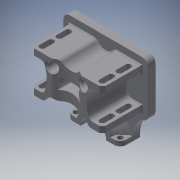
# Autodesk Inventor part: x-carriage
Saved by Autodesk Inventor 2018 (Build 220112000, 112)
## iProperties
Created: 2017-10-14
Part Number: x-carriage
Material: Generic
Document SubType Name: Modeling
Designer: Jurjen
Density: 1 g/cm^3
Appearance: Default
Author: Jurjen
Autodesk Inventor part; units mm, degrees
ref_plane "YZ Plane" through (0, 0, 0) normal (1, 0, 0) x (0, 1, 0)
ref_plane "XZ Plane" through (0, 0, 0) normal (0, 1, 0) x (-1, 0, 0)
ref_plane "XY Plane" through (0, 0, 0) normal (0, 0, 1) x (1, 0, 0)
sketch "Sketch1" plane through (0, 0, 0) normal (0, 0, 1) x (1, 0, 0)
  line L0 (-27, 20) -> (27, 20)
  line L1 (27, 20) -> (27, -15)
  line L2 (27, -15) -> (-27, -15)
  line L3 (-27, -15) -> (-27, 20)
  point P0 (0, 0)
  point P1 (0, 20)
  point P2 (-27, 2.5)
  dimension "d0" = 54
  dimension "d69" = 20
  dimension "d70" = 15
  constraints: 8 end point, 2 midpoint, 2 parallel, 1 horizontal, 1 perpendicular, 1 vertical alignment
  measures "d0" distance between parallel lines of L1 L3
  measures "d69" distance from line of L0 point (0, 0)
  measures "d70" distance from line of point (0, 0) L2
extrude "Extrusion1" add sketch "Sketch1" along normal mid plane 5
sketch "Sketch2" plane through (0, 0, 2.5) normal (0, 0, 1) x (1, 0, 0)
  circle A0 centre (10, 10) radius 1.6
  circle A1 centre (-10, 10) radius 1.6
  circle A2 centre (-10, -10) radius 1.6
  circle A3 centre (10, -10) radius 1.6
  line L0 (-10, 10) -> (10, 10) construction
  line L1 (-10, -10) -> (-10, 10) construction
  point P0 (0, 0)
  point P1 (0, 10)
  point P2 (-10, 0)
  dimension "d4" = 20
  dimension "d5" = 20
  dimension "d6" = 3.2
  constraints: 4 centre point, 4 end point, 3 equal radius, 3 horizontal alignment, 3 vertical alignment, 2 midpoint, 1 horizontal, 1 vertical
  measures "d4" distance of L0.end L0.start
  measures "d5" distance of L1.start L0.start
  measures "d6" diameter of A1
extrude "Extrusion2" cut sketch "Sketch2" against normal up to next
fillet "Fillet1" radius 4 4 edges at (-27, 20, 0) (-27, -15, 0) (27, -15, 0) (27, 20, 0)
sketch "Sketch3" plane through (0, 0, 2.5) normal (0, 0, 1) x (1, 0, 0)
  line L0 (-23, -15) -> (23, -15) projected
  arc A0 (8.15, -30) -> (-8.15, -30) centre (0, -30) ccw
  line L1 (17.15, -30) -> (8.15, -30)
  arc A1 (23, -15) -> (17.15, -30) centre (34.9437, -28.2988) ccw
  line L2 (0, -30) -> (0, 0) construction
  line L3 (-17.15, -30) -> (-8.15, -30)
  arc A2 (-17.15, -30) -> (-23, -15) centre (-34.9437, -28.2988) ccw
  dimension "d10" = 30
  dimension "d12" = 9
  dimension "d13" = 16.3
  constraints: 6 end point, 6 point on circle, 3 centre point, 3 symmetric about line, 1 horizontal, 1 horizontal alignment, 1 vertical, 1 vertical alignment, 1 other
  measures "d10" distance of L2.start L2.end
  measures "d12" distance of L1.start L1.end
  measures "d13" diameter of A0
extrude "Extrusion3" add sketch "Sketch3" against normal up to surface (5 mm away)
sketch "Sketch4" plane through (0, 0, 2.5) normal (0, 0, 1) x (1, 0, 0)
  arc A0 (8.15, -30) -> (-8.15, -30) centre (0, -30) ccw projected
  arc A1 (6.25, -30) -> (-6.25, -30) centre (0, -30) ccw
  line L0 (-6.25, -30) -> (-17.15, -30)
  arc A2 (-17.15, -30) -> (-23, -15) centre (-34.9437, -28.2988) ccw projected
  line L1 (17.15, -30) -> (8.15, -30) projected
  line L2 (17.15, -30) -> (6.25, -30)
  arc A3 (8.15, -30) -> (-8.15, -30) centre (0, -30) ccw
  point P0 (0, 0)
  dimension "d16" = 12.5
  constraints: 6 point on circle, 4 end point, 2 centre point, 2 coincident, 2 point on line, 1 collinear, 1 horizontal alignment
  measures "d16" diameter of A1
extrude "Extrusion4" add sketch "Sketch4" along normal blind 3.8 and the other way blind 1.8
sketch "Sketch5" plane through (0, 0, 2.5) normal (0, 0, 1) x (1, 0, 0)
  arc A0 (27, 16) -> (23, 20) centre (23, 16) ccw projected
  line L0 (23, 20) -> (-23, 20) projected
  arc A1 (-23, 20) -> (-27, 16) centre (-23, 16) ccw projected
  line L1 (-27, 16) -> (-27, -11) projected
  arc A2 (-27, -11) -> (-23, -15) centre (-23, -11) ccw projected
  arc A3 (-17.15, -30) -> (-23, -15) centre (-34.9437, -28.2988) ccw projected
  line L2 (-8.15, -30) -> (-17.15, -30) projected
  arc A4 (8.15, -30) -> (-8.15, -30) centre (0, -30) ccw projected
  line L3 (17.15, -30) -> (8.15, -30) projected
  arc A5 (23, -15) -> (17.15, -30) centre (34.9437, -28.2988) ccw projected
  arc A6 (23, -15) -> (27, -11) centre (23, -11) ccw projected
  line L4 (27, -11) -> (27, 16) projected
  circle A7 centre (-10, -10) radius 1.6 projected
  circle A8 centre (10, 10) radius 1.6 projected
  circle A9 centre (-10, 10) radius 1.6 projected
  circle A10 centre (10, -10) radius 1.6 projected
  arc A11 (23, -15) -> (17.15, -30) centre (34.9437, -28.2988) ccw projected
  line L5 (17.1161, -27) -> (7.5778, -27)
  line L6 (-7.5778, -27) -> (-17.1161, -27)
  point P0 (0, 0)
  dimension "d21" = 3
  constraints: 4 end point, 4 point on circle, 2 point on line, 1 horizontal
  measures "d21" distance between parallel lines of L3 L5
extrude "Extrusion5" add sketch "Sketch5" along normal up to surface (3.8 mm away) contours A5 L3 A4 L5 | A4 L2 A3 L6
sketch "Sketch6" plane through (0, 0, 6.3) normal (0, 0, 1) x (1, 0, 0)
  arc A0 (8.15, -30) -> (-8.15, -30) centre (0, -30) ccw projected
  arc A1 (8.15, -30) -> (-8.15, -30) centre (0, -30) ccw
  arc A2 (11.15, -30) -> (-11.15, -30) centre (0, -30) ccw
  arc A3 (6.25, -30) -> (-6.25, -30) centre (0, -30) ccw projected
  line L0 (-6.25, -30) -> (-17.15, -30) projected
  line L1 (-6.25, -30) -> (-17.15, -30)
  line L2 (6.25, -30) -> (12.2947, -30)
  point P0 (0, 0)
  dimension "d24" = 3
  constraints: 6 point on circle, 4 end point, 4 point on line, 2 centre point, 2 coincident, 2 horizontal
  measures "d24" radial gap between concentric circles of A2 A1
extrude "Extrusion6" add sketch "Sketch6" along normal blind 4 contours A0 L0 A2 L2
sketch "Sketch9" plane through (0, 0, 6.3) normal (0, 0, 1) x (1, 0, 0)
  arc A0 (-10.7388, -27) -> (-11.15, -30) centre (0, -30) ccw projected
  line L0 (-17.1161, -27) -> (-10.7388, -27) projected
  arc A1 (-17.15, -30) -> (-17.1161, -27) centre (-34.9437, -28.2988) ccw projected
  line L1 (-11.15, -30) -> (-17.15, -30) projected
  arc A2 (11.15, -30) -> (10.7388, -27) centre (0, -30) ccw projected
  line L2 (11.15, -30) -> (17.15, -30) projected
  arc A3 (17.1161, -27) -> (17.15, -30) centre (34.9437, -28.2988) ccw projected
  line L3 (10.7388, -27) -> (17.1161, -27) projected
  point P0 (0, 0)
extrude "Extrusion7" add sketch "Sketch9" along normal up to surface (4 mm away)
sketch "Sketch10" plane through (0, 0, 6.3) normal (0, 0, -1) x (-1, 0, 0)
  line L0 (10.7388, -27) -> (7.5778, -27) projected
  arc A0 (10.7388, -27) -> (-10.7388, -27) centre (0, -30) ccw projected
  line L1 (-7.5778, -27) -> (-10.7388, -27) projected
  arc A1 (7.5778, -27) -> (-7.5778, -27) centre (0, -30) ccw projected
  point P0 (0, 0)
extrude "Extrusion8" add sketch "Sketch10" along normal up to surface (3.8 mm away)
chamfer "Chamfer1" distance 5 angle 45 1 edges at (0, -18.85, 2.5)
fillet "Fillet2" radius 4 2 edges at (17.07, -28.5007, 10.3) (-17.07, -28.5007, 10.3)
fillet "Fillet3" radius 4 2 edges at (0, -18.85, 7.5) (0, -13.85, 2.5)
sketch "Sketch13" plane through (-17.15, -30, -2.5) normal (0, -1, 0) x (1, 0, 0)
  circle A0 centre (3, 9.8) radius 1.6
  circle A1 centre (31.3, 9.8) radius 1.6
  line L0 (0, 0) -> (0, 8.8) projected
  line L1 (9, 12.8) -> (4.0149, 12.8) projected
  line L2 (34.3, 8.8) -> (34.3, 0) projected
  point P0 (17.15, 2.5)
  dimension "d45" = 3.2
  dimension "d46" = 3
  dimension "d47" = 3
  dimension "d48" = 3
  constraints: 2 centre point, 1 equal radius, 1 horizontal alignment
  measures "d45" diameter of A0
  measures "d46" distance from line of A0.centre L0
  measures "d47" distance from line of L1 A0.centre
  measures "d48" distance from line of A1.centre L2
extrude "Extrusion10" cut sketch "Sketch13" against normal up to next
sketch "Sketch17" plane through (0, 0, 2.5) normal (0, 0, 1) x (1, 0, 0)
  line L0 (-13.1229, -10.9) -> (-23, -10.9)
  line L1 (-23, -10.9) -> (-23, -6.9)
  line L2 (-23, -6.9) -> (-14, -6.9)
  line L3 (-14, -6.9) -> (-14, -4.9)
  line L4 (-14, 11.2) -> (-23, 11.2)
  circle A0 centre (-10, 10) radius 1.6 projected
  circle A1 centre (-10, 10) radius 3
  circle A2 centre (-10, -10) radius 1.6 projected
  arc A3 (-7.3604, -8.104) -> (-13.1229, -10.9) centre (-10, -10) ccw
  line L5 (-23, 15.2) -> (-6, 15.2)
  line L6 (-23, 11.2) -> (-23, 15.2)
  line L7 (0, 0) -> (0, 11.3763) construction
  arc A4 (-6, 15.2) -> (0, 11.3763) centre (-0.0763, 17.8758) ccw
  arc A5 (0, -6.9) -> (-7.3604, -8.104) centre (0, -30) ccw
  line L8 (0, -6.9) -> (0, 0) construction
  arc A6 (-7, -1.7545) -> (-7, 6.0545) centre (-14.1224, 2.15) ccw
  arc A7 (0, -0.9) -> (-7, -1.7545) centre (0, -30) ccw
  line L9 (13.1229, -10.9) -> (23, -10.9)
  line L10 (23, -10.9) -> (23, -6.9)
  line L11 (23, -6.9) -> (14, -6.9)
  line L12 (14, 11.2) -> (23, 11.2)
  circle A8 centre (10, 10) radius 3
  arc A9 (13.1229, -10.9) -> (7.3604, -8.104) centre (10, -10) ccw
  line L13 (23, 15.2) -> (6, 15.2)
  line L14 (23, 11.2) -> (23, 15.2)
  arc A10 (0, 11.3763) -> (6, 15.2) centre (0.0763, 17.8758) ccw
  arc A11 (7.3604, -8.104) -> (0, -6.9) centre (0, -30) ccw
  arc A12 (7, 6.0545) -> (7, -1.7545) centre (14.1224, 2.15) ccw
  arc A13 (7, -1.7545) -> (0, -0.9) centre (0, -30) ccw
  arc A14 (14.6749, -27) -> (-14.6749, -27) centre (0, -30) ccw projected
  arc A15 (-7, 6.0545) -> (0, 4.9807) centre (0.8793, 34.0674) ccw
  arc A16 (0, 4.9807) -> (7, 6.0545) centre (-0.8793, 34.0674) ccw
  arc A17 (-14, -4.9) -> (-14, 9.2) centre (-32.7162, 2.15) ccw
  arc A18 (14, 9.2) -> (14, -4.9) centre (32.7162, 2.15) ccw
  line L15 (14, -6.9) -> (14, -4.9)
  line L16 (14, 9.2) -> (14, 11.2)
  line L17 (-14, 9.2) -> (-14, 11.2)
  line L18 (-14, -4.9) -> (-14, 9.2) construction
  point P0 (0, 8.6643)
  point P1 (-14, 2.15)
  point P2 (-6, 2.15)
  point P3 (-12.7162, 2.15)
  dimension "d71" = 6
  dimension "d72" = 6.5
  dimension "d73" = 4
  dimension "d75" = 4
  dimension "d76" = 17
  dimension "d77" = 18.1
  dimension "d78" = 14
  dimension "d80" = 6.5
  dimension "d81" = 9
  dimension "d82" = 11.2
  dimension "d98" = 6
  dimension "d99" = 6
  dimension "d100" = 7
  dimension "d103" = 29.1
  dimension "d104" = 20
  dimension "d105" = 2
  dimension "d106" = 2
  constraints: 38 end point, 30 point on circle, 22 symmetric about line, 16 centre point, 9 perpendicular, 5 point on line, 3 vertical, 3 vertical alignment, 2 coincident, 2 concentric, 2 horizontal alignment, 8 other
  measures "d71" diameter of A1
  measures "d72" diameter of A3
  measures "d73" distance between parallel lines of L0 L2
  measures "d75" distance between parallel lines of L5 L4
  measures "d76" distance of L5.start L5.end
  measures "d77" distance of L2.end L4.start
  measures "d78" distance from line of L7.start L3
  measures "d80" radius of A4
  measures "d81" distance between parallel lines of L6 L3
  measures "d82" distance from line of L7.start L4
  measures "d98" distance of L8.start A7.start
  measures "d99" distance from line of L7 point (-6, 2.15)
  measures "d100" distance from line of L7 A6.end
  measures "d103" radius of A15
  measures "d104" radius of A17
  measures "d105" distance of L2.end L3.end
  measures "d106" distance of L4.start L17.start
extrude "Extrusion13" add sketch "Sketch17" along normal blind 25 contours L0 L1 L2 L3 A17 L17 L4 L6 L5 A4 A10 L13 L14 L12 L16 A18 L15 L11 L10 L9 A9 A11 A5 A3
fillet "Fillet6" radius 3 13 edges at (-14, 11.2, 15) (-14, 9.2, 15) (-14, -4.9, 15) (-14, -6.9, 15) (6, 15.2, 15) (-6, 15.2, 15) (-7.3604, -8.104, 15) (7.3604, -8.104, 15) (13.1229, -10.9, 15) (-13.1229, -10.9, 15) (14, 11.2, 15) (14, -4.9, 15) (14, -6.9, 15)
sketch "Sketch18" plane through (-23, -10.9, 2.5) normal (0, -1, 0) x (1, 0, 0)
  line L0 (7.1134, 25) -> (7.1134, 0) projected
  line L1 (0, 25) -> (7.1134, 25) projected
  line L2 (0, 0) -> (0, 25) projected
  line L3 (7.1134, 0) -> (0, 0) projected
  line L4 (2, 23) -> (5.5, 23)
  line L5 (5.5, 23) -> (5.5, 14)
  line L6 (5.5, 14) -> (2, 14)
  line L7 (2, 14) -> (2, 23)
  line L8 (2, 12) -> (5.5, 12)
  line L9 (5.5, 12) -> (5.5, 3)
  line L10 (5.5, 3) -> (2, 3)
  line L11 (2, 3) -> (2, 12)
  point P0 (23, -2.5)
  dimension "d110" = 3.5
  dimension "d111" = 2
  dimension "d112" = 2
  dimension "d113" = 9
  dimension "d114" = 2
  dimension "d115" = 9
  constraints: 16 end point, 4 parallel, 2 horizontal, 2 perpendicular, 2 vertical alignment, 1 point on line
  measures "d110" distance of L4.start L4.end
  measures "d111" distance between parallel lines of L2 L7
  measures "d112" distance between parallel lines of L1 L4
  measures "d113" distance between parallel lines of L4 L6
  measures "d114" distance between parallel lines of L6 L8
  measures "d115" distance between parallel lines of L10 L8
extrude "Extrusion14" cut sketch "Sketch18" against normal through all contours L4 L5 L6 L7 | L8 L9 L10 L11
chamfer "Chamfer2" distance 1 angle 45 16 edges at (-17.5, -8.9, 25.5) (-21, -8.9, 25.5) (-17.5, -8.9, 14.5) (-21, -8.9, 14.5) (-21, -8.9, 5.5) (-21, -8.9, 16.5) (-17.5, -8.9, 5.5) (-17.5, -8.9, 16.5) (-17.5, 13.2, 16.5) (-17.5, 13.2, 5.5) (-17.5, 13.2, 14.5) (-17.5, 13.2, 25.5) (-21, 13.2, 5.5) (-21, 13.2, 16.5) (-21, 13.2, 25.5) (-21, 13.2, 14.5)
mirror "Mirror2" about plane through (0, 0, 0) normal (1, 0, 0) of "Extrusion14", "Chamfer2"
chamfer "Chamfer4" distance 2 angle 45 4 edges at (23, -8.9, 27.5) (23, 13.2, 27.5) (-23, -8.9, 27.5) (-23, 13.2, 27.5)
chamfer "Chamfer5" distance 0.7 angle 45 32 edges at (-19.4433, -10.9, 2.5) (-14.1581, -10.3519, 2.5) (-11.0447, -6.9225, 2.5) (-7.0827, -7.7127, 2.5) (0, -6.9, 2.5) (7.0827, -7.7127, 2.5) (11.0447, -6.9225, 2.5) (14.1581, -10.3519, 2.5) (19.4433, -10.9, 2.5) (-23, -8.9, 2.5) (-19.9142, -6.9, 2.5) (-15.1035, -6.3545, 2.5) (-13.9989, -4.8974, 2.5) (-12.7162, 2.15, 2.5) (-13.9989, 9.1974, 2.5) (-15.1035, 10.6545, 2.5) (-19.9142, 11.2, 2.5) (-15.3472, 15.2, 2.5) (-6.3485, 14.8811, 2.5) (-2.9583, 12.0497, 2.5) (-23, 13.2, 2.5) (15.3472, 15.2, 2.5) (6.3485, 14.8811, 2.5) (2.9583, 12.0497, 2.5) (12.7162, 2.1615, 2.5) (13.9989, -4.8974, 2.5) (15.1035, -6.3545, 2.5) (19.9142, -6.9, 2.5) (15.0964, 10.6495, 2.5) (19.9142, 11.2, 2.5) (23, 13.2, 2.5) (23, -8.9, 2.5)
sketch "Sketch19" plane through (-21, -10.9, 27.5) normal (0, -1, 0) x (1, 0, 0)
  line L0 (0, 0) -> (4.1716, 0) projected
  line L1 (7.0081, 0) -> (4.1716, 0) projected
  line L2 (7.0081, 0) -> (7.0081, 0) projected
  line L3 (7.0081, 0) -> (7.0081, 0) projected
  line L4 (6.9941, 0) -> (7.0081, 0) projected
  line L5 (4.1716, 0) -> (6.9941, 0) projected
  line L6 (4.1716, 0) -> (0, 0) projected
  line L7 (0, 0) -> (5.1134, 0) projected
  line L8 (7.9389, 0) -> (5.1134, 0) projected
  line L9 (7.9389, 0) -> (12.7637, 0) projected
  line L10 (15.1514, 0) -> (12.7637, 0) projected
  line L11 (15.1514, 0) -> (26.8486, 0) projected
  line L12 (29.2363, 0) -> (26.8486, 0) projected
  line L13 (29.2363, 0) -> (34.0611, 0) projected
  line L14 (36.8866, 0) -> (34.0611, 0) projected
  line L15 (36.8866, 0) -> (42, 0) projected
  line L16 (42, 0) -> (37.8284, 0) projected
  line L17 (35.0059, 0) -> (37.8284, 0) projected
  line L18 (34.9919, 0) -> (35.0059, 0) projected
  line L19 (34.9919, 0) -> (35, 0) projected
  line L20 (37.8284, 0) -> (35, 0) projected
  line L21 (37.8284, 0) -> (42, 0) projected
  line L22 (42, 0) -> (28.6944, 0) projected
  line L23 (26.2887, 0) -> (28.6944, 0) projected
  line L24 (26.2887, 0) -> (21, 0) projected
  line L25 (21, 0) -> (15.7113, 0) projected
  line L26 (13.3056, 0) -> (15.7113, 0) projected
  line L27 (13.3056, 0) -> (0, 0) construction
  line L28 (14, 0) -> (21, 0) projected
  line L29 (21, 0) -> (28, 0) projected
  line L30 (28, 0) -> (28, 0) projected
  line L31 (28, 0) -> (14, 0) projected
  line L32 (14, 0) -> (14, 0) projected
  arc A0 (11.7122, 0) -> (30.2878, 0) centre (21, 11.7786) ccw
  line L33 (11.7122, 0) -> (30.2878, 0)
  line L34 (7.0081, 0) -> (4.1716, 0) projected
  point P0 (21, -27.5)
  point P1 (15, 0)
  point P2 (7, 0)
  point P3 (27, 0)
  point P4 (21, -3.2214)
  dimension "d130" = 15
  constraints: 3 point on circle, 2 end point, 1 centre point, 1 collinear, 1 midpoint, 1 point on line, 1 vertical alignment
  measures "d130" radius of A0
extrude "Extrusion15" cut sketch "Sketch19" against normal blind 40
chamfer "Chamfer6" distance 0.7 angle 45 6 edges at (-7.6437, 11.8568, 26.3723) (-7.6437, 8.1432, 26.3723) (-13, 10, 27.5) (7, 10, 26.0121) (11.8525, 7.6403, 27.5) (11.8525, 12.3597, 27.5)
fillet "Fillet7" radius 3 8 edges at (-9.2878, -0.2299, 27.5) (-9.2878, 14.4154, 27.5) (-9.3911, 13.2843, 27.1403) (9.2878, 14.4154, 27.5) (9.3912, 13.2839, 27.1399) (9.2878, -0.2299, 27.5) (9.3912, 6.7161, 27.1399) (-9.3911, 6.7157, 27.1403)
sketch "Sketch14" plane through (0, 0, 2.5) normal (0, 0, 1) x (1, 0, 0)
  line L0 (19.5, 6.65) -> (-19.5, 6.65)
  line L1 (-19.5, 6.65) -> (-19.5, 2.65)
  line L2 (-19.5, 2.65) -> (-6.5, 2.65)
  line L3 (-6.5, 2.65) -> (-6.5, -2.65)
  line L4 (-6.5, -2.65) -> (-19.5, -2.65)
  line L5 (-19.5, -2.65) -> (-19.5, -6.65)
  line L6 (-19.5, -6.65) -> (19.5, -6.65)
  line L7 (19.5, -6.65) -> (19.5, -2.65)
  line L8 (19.5, -2.65) -> (6.5, -2.65)
  line L9 (6.5, -2.65) -> (6.5, 2.65)
  line L10 (6.5, 2.65) -> (19.5, 2.65)
  line L11 (19.5, 6.65) -> (19.5, 2.65)
  point P0 (0, 0)
  point P1 (0, 6.65)
  point P2 (0, -6.65)
  point P3 (6.5, 0)
  point P4 (-6.5, 0)
  dimension "d51" = 4
  dimension "d52" = 4
  dimension "d53" = 5.3
  dimension "d54" = 13
  dimension "d55" = 39
  dimension "d56" = 13
  constraints: 24 end point, 9 perpendicular, 5 point on line, 4 midpoint, 2 horizontal alignment, 2 vertical alignment, 1 horizontal
  measures "d51" distance between parallel lines of L10 L0
  measures "d52" distance between parallel lines of L6 L8
  measures "d53" distance between parallel lines of L8 L10
  measures "d54" distance between parallel lines of L9 L11
  measures "d55" distance between parallel lines of L1 L11
  measures "d56" distance between parallel lines of L1 L3
sketch "Sketch15" plane through (-19.5, -6.65, 2.5) normal (0, -1, 0) x (1, 0, 0)
  line L0 (4, 21.5) -> (8, 21.5)
  line L1 (8, 21.5) -> (8, 13.5)
  line L2 (8, 13.5) -> (4, 13.5)
  line L3 (4, 13.5) -> (4, 21.5)
  line L4 (4, 11) -> (8, 11)
  line L5 (8, 11) -> (8, 3)
  line L6 (8, 3) -> (4, 3)
  line L7 (4, 3) -> (4, 11)
  line L8 (0, 25) -> (39, 25) projected
  line L9 (0, 0) -> (0, 25) projected
  point P0 (19.5, -2.5)
  dimension "d59" = 4
  dimension "d60" = 8
  dimension "d61" = 8
  dimension "d62" = 3.5
  dimension "d63" = 2.5
  dimension "d64" = 4
  constraints: 16 end point, 4 parallel, 2 horizontal, 2 perpendicular, 1 point on line, 1 vertical alignment
  measures "d59" distance between parallel lines of L1 L3
  measures "d60" distance between parallel lines of L0 L2
  measures "d61" distance between parallel lines of L6 L4
  measures "d62" distance between parallel lines of L8 L0
  measures "d63" distance between parallel lines of L4 L2
  measures "d64" distance between parallel lines of L9 L3
body "Solid1"
